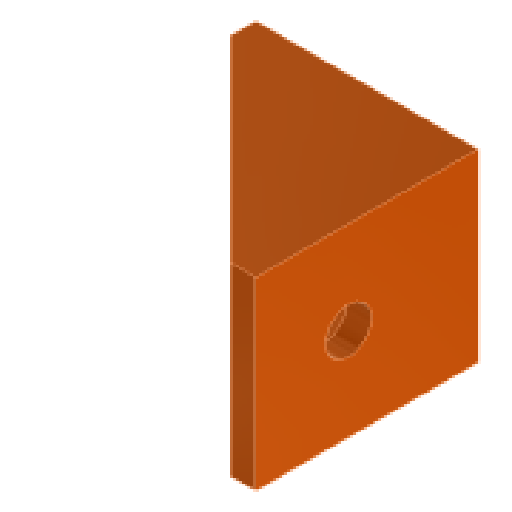
# Autodesk Inventor part: Beam_CornerTri
Saved by Autodesk Inventor 2023.2 (Build 272271000, 271)
## iProperties
Created: 2020-05-08
Part Number: Beam_CornerTri
Material: ABS Plastic
Document SubType Name: Modeling
Designer: Remo
Density: 1.06 g/cm^3
Appearance: Smooth - Light Orange
Description: 3DP Part / PET-G / Beam Corner Triangle
Mass: 1.71401 g
Surface Area: 16.8462 cm^2
Volume: 1.61699 cm^3
Author: Remo
Revision Number: 2
Autodesk Inventor part; units mm, degrees
ref_plane "YZ Plane" through (0, 0, 0) normal (1, 0, 0) x (0, 1, 0)
ref_plane "XZ Plane" through (0, 0, 0) normal (0, 1, 0) x (-1, 0, 0)
ref_plane "XY Plane" through (0, 0, 0) normal (0, 0, 1) x (1, 0, 0)
sketch "Sketch1" plane through (0, 0, 0) normal (0, 0, 1) x (1, 0, 0)
  line L0 (0, 0) -> (0, -18)
  line L1 (0, -18) -> (-2, -18)
  line L2 (-2, -18) -> (-18, -2)
  line L3 (-18, -2) -> (-18, 0)
  line L4 (-18, 0) -> (0, 0)
  dimension "d0" = 18
  dimension "d1" = 2
  constraints: 10 end point, 4 perpendicular, 1 parallel, 1 vertical
  measures "d0" distance of L3.end L0.start
  measures "d1" distance of L2.end L3.end
extrude "Extrusion1" add sketch "Sketch1" along normal blind 2.5
sketch "Sketch2" plane through (0, 0, 2.5) normal (0, 0, 1) x (1, 0, 0)
  line L0 (0, -18) -> (0, 0) projected
  line L1 (0, 0) -> (-18, 0) projected
  line L2 (-18, 0) -> (-18, -2) projected
  line L3 (-18, -2) -> (-2, -18) projected
  line L4 (-2, -18) -> (0, -18) projected
  line L5 (-18, 0) -> (-18, -2) projected
  line L6 (-18, -2) -> (-2, -2)
  line L7 (-2, -18) -> (0, -18) projected
  line L8 (-2, -2) -> (-2, -18)
  constraints: 4 end point, 1 horizontal, 1 perpendicular
extrude "Extrusion2" add sketch "Sketch2" along normal blind 10 contours L4 L8 L6 L2 L1 L0
sketch "Sketch3" plane through (0, 0, 12.5) normal (0, 0, 1) x (1, 0, 0)
  line L0 (-2, -2) -> (-18, -2) projected
  line L1 (-18, -2) -> (-2, -18) projected
  line L2 (-2, -18) -> (-2, -2) projected
  line L3 (0, -18) -> (0, 0) projected
  line L4 (0, 0) -> (-18, 0) projected
  line L5 (-18, 0) -> (-18, -2) projected
  line L6 (-18, -2) -> (-2, -2) projected
  line L7 (-2, -2) -> (-2, -18) projected
  line L8 (-2, -18) -> (0, -18) projected
extrude "Extrusion3" add sketch "Sketch3" along normal blind 2.5
sketch "Sketch4" plane through (-18, 0, 0) normal (0, 1, 0) x (1, 0, 0)
  line L0 (0, 0) -> (18, 0) projected
  line L1 (0, 0) -> (0, -15) projected
  line L2 (18, -15) -> (0, -15) projected
  line L3 (18, 0) -> (18, -15) projected
  point P0 (7.5, -7.5)
  dimension "d8" = 7.5
  dimension "d9" = 7.5
  measures "d8" distance from line of L1 point (7.5, -7.5)
  measures "d9" distance from line of L0 point (7.5, -7.5)
hole "Hole1" at (-10.5, 0, 7.5) direction (0, -1, 0) diameter 3.7 depth 8 tip angle 118
sketch "Sketch5" plane through (0, -18, 0) normal (1, 0, 0) x (0, 0, -1)
  line L0 (0, 18) -> (0, 0) projected
  line L1 (0, 18) -> (-15, 18) projected
  line L2 (-15, 0) -> (-15, 18) projected
  line L3 (0, 0) -> (-15, 0) projected
  point P0 (-7.5, 7.5)
  dimension "d17" = 7.5
  dimension "d18" = 7.5
  measures "d17" distance from line of L2 point (-7.5, 7.5)
  measures "d18" distance from line of L3 point (-7.5, 7.5)
hole "Hole2" at (0, -10.5, 7.5) direction (-1, 0, 0) diameter 3.7 depth 8 tip angle 118
equation "\"d9\" = d8"
body "Solid1"
